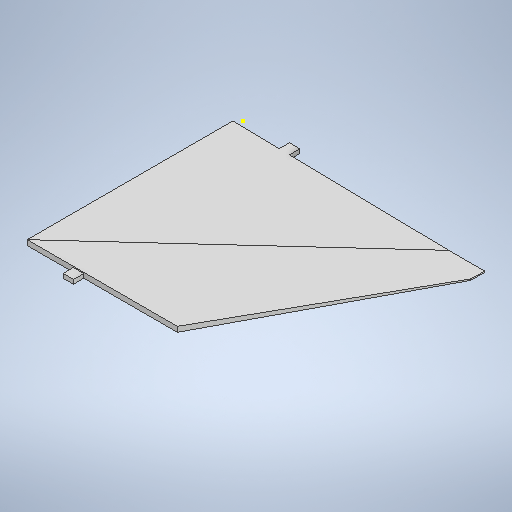
# Autodesk Inventor part: 坂
Saved by Autodesk Inventor 2026.2 (Build 302298010, 298A)
## iProperties
Created: 2026-05-25
Part Number: 坂
Material: 一般
Document SubType Name: Modeling
Designer: Yagis
Density: 1 g/cm^3
Appearance: 既定
Author: Yagis
Autodesk Inventor part; units mm, degrees
ref_plane "YZ Plane" through (0, 0, 0) normal (1, 0, 0) x (0, 1, 0)
ref_plane "XZ Plane" through (0, 0, 0) normal (0, 1, 0) x (-1, 0, 0)
ref_plane "XY Plane" through (0, 0, 0) normal (0, 0, 1) x (1, 0, 0)
sketch "スケッチ1" plane through (0, 0, 0) normal (0, 1, 0) x (-1, 0, 0)
  point P0 (0, 0)
sketch "スケッチ2" plane through (0, 0, 0) normal (0, 0, 1) x (1, 0, 0)
  line L0 (0, 0) -> (0, 5)
  line L1 (0, 5) -> (210, 1)
  line L2 (0, 0) -> (210, 0)
  line L3 (210, 1) -> (210, 0)
  dimension "d0" = 5
  dimension "d1" = 210
  dimension "d28" = 1
  constraints: 8 end point, 2 vertical, 1 horizontal
  measures "d0" distance of L0.start L0.end
  measures "d1" distance of L2.end L0.start
  measures "d28" distance of L1.end L2.end
extrude "押し出し1" add sketch "スケッチ2" along normal blind 220
sketch "スケッチ4" plane through (0, 0, 220) normal (0, 0, 1) x (1, 0, 0)
  line L0 (0, 5) -> (0, 0) projected
  line L1 (55, 0) -> (245, 0)
  line L2 (245, 0) -> (245, 5)
  line L3 (245, 5) -> (55, 5)
  line L4 (55, 5) -> (55, 0)
  line L5 (0, 5) -> (45, 5)
  line L6 (45, 5) -> (45, 0)
  line L7 (45, 0) -> (0, 0)
  line L8 (0, 0) -> (0, 5)
  point P0 (0, 0)
  dimension "d8" = 5
  dimension "d9" = 190
  dimension "d10" = 55
  dimension "d23" = 45
  dimension "d30" = 5
  constraints: 16 end point, 4 parallel, 2 horizontal, 2 perpendicular
  measures "d8" distance between parallel lines of L1 L3
  measures "d9" distance between parallel lines of L2 L4
  measures "d10" distance between parallel lines of L0 L4
  measures "d23" distance of L6.end L7.end
  measures "d30" distance of L5.end L6.end
extrude "押し出し2" cut sketch "スケッチ4" against normal blind 10
sketch "スケッチ5" plane through (0, 0, 0) normal (0, 0, -1) x (-1, 0, 0)
  line L0 (-55, 0) -> (-245, 0)
  line L1 (-245, 0) -> (-245, 4)
  line L2 (-245, 4) -> (-55, 4)
  line L3 (-55, 4) -> (-55, 0)
  line L4 (0, 5) -> (0, 0) projected
  line L5 (0, 5) -> (-45, 5)
  line L6 (-45, 5) -> (-45, 0)
  line L7 (-45, 0) -> (0, 0)
  line L8 (0, 0) -> (0, 5)
  dimension "d13" = 4
  dimension "d14" = 55
  dimension "d15" = 190
  dimension "d22" = 45
  dimension "d29" = 5
  constraints: 16 end point, 4 parallel, 2 horizontal, 2 perpendicular
  measures "d13" distance between parallel lines of L2 L0
  measures "d14" distance between parallel lines of L4 L3
  measures "d15" distance of L0.start L0.end
  measures "d22" distance between parallel lines of L6 L4
  measures "d29" distance between parallel lines of L7 L5
extrude "押し出し3" cut sketch "スケッチ5" against normal blind 10
sketch "スケッチ7" plane through (0, 0, 10) normal (-1, 0, 0) x (0, 0, 1)
  line L0 (200, 0) -> (200, 5)
  line L1 (200, 5) -> (0, 1)
  line L2 (0, 0) -> (200, 0)
  line L3 (0, 1) -> (0, 0)
  point P0 (-10, 0)
  dimension "d24" = 5
  dimension "d27" = 200
  dimension "d31" = 1
  constraints: 8 end point, 2 perpendicular, 1 coincident, 1 vertical
  measures "d24" distance of L0.start L0.end
  measures "d27" distance from line of L2.start L0
  measures "d31" distance of L1.end L2.start
extrude "押し出し5" add sketch "スケッチ7" against normal blind 245
sketch "スケッチ6" plane through (0, 0, 0) normal (0, -1, 0) x (1, 0, 0)
  line L0 (0, 0) -> (0, 220) projected
  line L1 (55, 10) -> (210, 10) projected
  line L2 (245, 23.5) -> (146, 210)
  line L3 (245, 210) -> (245, 23.5)
  line L4 (146, 210) -> (245, 23.5)
  line L5 (146, 210) -> (245, 210)
  line L6 (210, 210) -> (55, 210) projected
  point P0 (235, 210)
  point P1 (235, 10)
  dimension "d18" = 146
  dimension "d19" = 13.5
  constraints: 8 end point, 1 collinear, 1 horizontal, 1 vertical
  measures "d18" distance from line of L0 L2.end
  measures "d19" distance from line of L1 L2.start
extrude "押し出し4" cut sketch "スケッチ6" against normal blind 10
